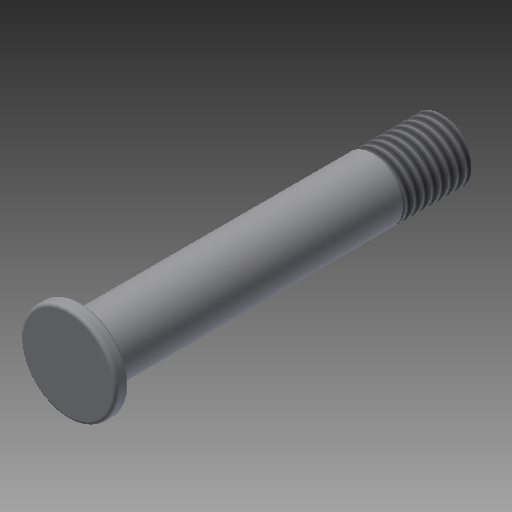
# Autodesk Inventor part: Kingpin
Saved by Autodesk Inventor 2019 (Build 230136000, 136)
## iProperties
Created: 2011-09-21
Part Number: Kingpin
Document SubType Name: Modeling
Designer: Stefano
Density: 1 g/cm^3
Material: 一般
Appearance: 既定
Author: Stefano
Autodesk Inventor part; units mm, degrees
ref_plane "YZ Plane" through (0, 0, 0) normal (1, 0, 0) x (0, 1, 0)
ref_plane "XZ Plane" through (0, 0, 0) normal (0, 1, 0) x (-1, 0, 0)
ref_plane "XY Plane" through (0, 0, 0) normal (0, 0, 1) x (1, 0, 0)
sketch "Schizzo1" plane through (0, 0, 0) normal (0, 0, 1) x (1, 0, 0)
  circle A0 centre (0, 0) radius 4.5
  dimension "d0" = 9
  constraints: 1 centre point, 1 coincident
  measures "d0" diameter of A0
extrude "Estrusione1" add sketch "Schizzo1" along normal mid plane 53
sketch "Schizzo2" plane through (0, 0, 26.5) normal (0, 0, 1) x (1, 0, 0)
  circle A0 centre (0, 0) radius 4.5 projected
  circle A1 centre (0, 0) radius 7
  dimension "d3" = 14
  constraints: 1 centre point, 1 coincident
  measures "d3" diameter of A1
extrude "Estrusione2" add sketch "Schizzo2" along normal blind 2 contours A0 | A1
chamfer "Smusso1" distance 0.5 angle 45 1 edges at (-4.5, 0, -26.5)
thread "Filettatura1" size "M9x1.25" class "6g" standard "ANSI Metric M Profile" length 10
fillet "Raccordo1" radius 0.5 2 edges at (-7, 0, 28.5) (-7, 0, 26.5)
